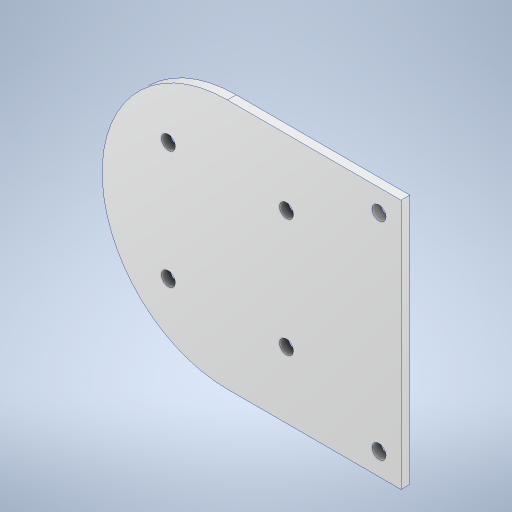
# Autodesk Inventor part: link4_plate2
Saved by Autodesk Inventor 2024 (Build 280153000, 153)
## iProperties
Created: 2024-12-13
Part Number: link4_plate2
Material: アルミニウム 6061
Document SubType Name: Modeling
Designer: hirek
Density: 2.7 g/cm^3
Appearance: アルミニウム - フラット
Mass: 15.4015 g
Surface Area: 62.3196 cm^2
Volume: 5.70425 cm^3
Author: hirek
Autodesk Inventor part; units mm, degrees
ref_plane "YZ Plane" through (0, 0, 0) normal (1, 0, 0) x (0, 1, 0)
ref_plane "XZ Plane" through (0, 0, 0) normal (0, 1, 0) x (-1, 0, 0)
ref_plane "XY Plane" through (0, 0, 0) normal (0, 0, 1) x (1, 0, 0)
sketch "スケッチ1" plane through (0, 0, 0) normal (0, 0, 1) x (1, 0, 0)
  circle A0 centre (0, 0) radius 28.5
  line L0 (0, 28.5) -> (39.5, 28.5)
  line L1 (39.5, 28.5) -> (39.5, -28.5)
  line L2 (39.5, -28.5) -> (0, -28.5)
  line L3 (0, -28.5) -> (0, 28.5)
  point P0 (28.5, 0)
  dimension "d0" = 57
  dimension "d19" = 39.5
  constraints: 8 end point, 2 parallel, 1 coincident, 1 horizontal, 1 midpoint, 1 perpendicular, 3 other
  measures "d19" distance from line of L1 point (0, 0)
extrude "押し出し1" add sketch "スケッチ1" along normal blind 2
sketch "スケッチ3" plane through (0, 0, 2) normal (0, 0, 1) x (1, 0, 0)
  circle A0 centre (0, 0) radius 19
  line L0 (0, 0) -> (13.435, -13.435)
  line L1 (0, 0) -> (19, 0) construction
  line L2 (39.5, 28.5) -> (0, 28.5) projected
  line L3 (34.5, 28.5) -> (34.5, -28.5)
  line L4 (0, -28.5) -> (39.5, -28.5) projected
  line L5 (39.5, -28.5) -> (39.5, 28.5) projected
  point P0 (13.435, 13.435)
  point P1 (-13.435, 13.435)
  point P2 (-13.435, -13.435)
  point P3 (34.5, 23.5)
  point P4 (34.5, -23.5)
  dimension "d22" = 38
  dimension "d23" = 45
  dimension "d26" = 360
  dimension "d28" = 5
  dimension "d29" = 5
  dimension "d37" = 5
  constraints: 6 end point, 4 point on line, 2 coincident, 1 equal length, 1 horizontal, 1 vertical, 8 other
  measures "d23" angle of L0 L1
  measures "d28" distance from line of point (34.5, 23.5) L2
  measures "d29" distance from line of L4 point (34.5, -23.5)
  measures "d37" distance between parallel lines of L5 L3
hole "穴2" at (13.435, -13.435, 2) at (13.435, 13.435, 2) at (-13.435, 13.435, 2) at (-13.435, -13.435, 2) at (34.5, 23.5, 2) at (34.5, -23.5, 2) direction (0, 0, -1) diameter 3.2 end through all
